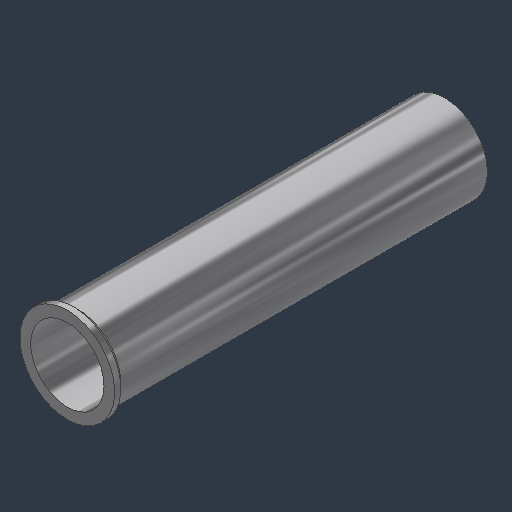
# Autodesk Inventor part: TUBE,1.5IN,ARM
Saved by Autodesk Inventor 2024.3 (Build 283343000, 343)
## iProperties
ILogicPurgeVersion: 0.0.0.0
OnSaveVersion: 3.5.0.0
OnSaveAssembly: COREAutomationManager
Category: _
Manager: _
Created: 2025-03-10
Part Number: TUBE,1.5IN,ARM
Checked By: 00
Engr Approved By: _
User Status: Work In Process
Material: Aluminum 7075
Description: STANDARD (mm)
Document SubType Name: Modeling
Mfg Approved By: John.Thibert
Designer: John.Thibert
Manufacturer: Standard
Standards Organization: Custom
Mass: 235.251 g
Surface Area: 527.669 cm^2
Volume: 83.7192 cm^3
Density: 2.81 g/cm^3
Appearance: Aluminum - Polished
CN_MASS: 0.21
CN_SERVICEABLE: _
FIRST_DESCRIPTION: _
SECOND_DESCRIPTION: _
THIRD_DESCRIPTION: _
ModelCat: Uncategorized
MaterialName: Aluminum 7075
Subject: _
Author: John.Thibert
Keywords: -
Revision Number: A
Autodesk Inventor part; units mm, degrees
ref_plane "YZ Plane" through (0, 0, 0) normal (1, 0, 0) x (0, 1, 0)
ref_plane "XZ Plane" through (0, 0, 0) normal (0, 1, 0) x (-1, 0, 0)
ref_plane "XY Plane" through (0, 0, 0) normal (0, 0, 1) x (1, 0, 0)
sketch "Sketch2" plane through (0, 0, 0) normal (0, 0, 1) x (1, 0, 0)
  circle A0 centre (0, 0) radius 19.05
  circle A1 centre (0, 0) radius 22.225
  dimension "d0" = 38.1
  dimension "d1" = 3.175
  constraints: 2 centre point, 1 coincident
  measures "d0" diameter of A0
  measures "d1" radial gap between concentric circles of A0 A1
extrude "Extrusion1" add sketch "Sketch2" along normal mid plane 195.98
sketch "Sketch3" plane through (0, 0, 97.99) normal (0, 0, -1) x (-1, 0, 0)
  circle A0 centre (0, 0) radius 22.225 projected
  circle A1 centre (0, 0) radius 24.6
  dimension "d4" = 49.2
  dimension "d7" = 2.375
  constraints: 1 centre point
  measures "d4" diameter of A1
  measures "d7" radial gap between concentric circles of A1 A0
extrude "Extrusion2" add sketch "Sketch3" along normal blind 3.175
chamfer "Chamfer2" distance 2.3749 angle 45 1 edges at (-22.225, 0, 94.815)
body "Solid1"
